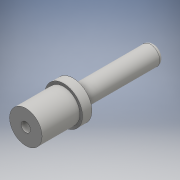
# Autodesk Inventor part: driven_shaft
Saved by Autodesk Inventor 2016 (Build 200138000, 138)
## iProperties
Created: 2015-10-28
Part Number: driven_shaft
Material: Gold
Document SubType Name: Modeling
Designer: Meet
Density: 19.3 g/cm^3
Appearance: Metal 1600F Hot
Author: Meet
Autodesk Inventor part; units mm, degrees
ref_plane "YZ Plane" through (0, 0, 0) normal (1, 0, 0) x (0, 1, 0)
ref_plane "XZ Plane" through (0, 0, 0) normal (0, 1, 0) x (-1, 0, 0)
ref_plane "XY Plane" through (0, 0, 0) normal (0, 0, 1) x (1, 0, 0)
sketch "Sketch1" plane through (0, 0, 0) normal (0, 1, 0) x (-1, 0, 0)
  circle A0 centre (0, 0) radius 10
  circle A1 centre (0, 0) radius 8.6
  constraints: 2 centre point, 2 coincident
extrude "Extrusion1" add sketch "Sketch1" along normal blind 5 contours A0 | A1
sketch "Sketch2" plane through (0, 0, 0) normal (0, -1, 0) x (1, 0, 0)
  circle A0 centre (0, 0) radius 8.6
  circle A1 centre (0, 0) radius 2.5
  constraints: 2 centre point, 2 coincident
extrude "Extrusion2" add sketch "Sketch2" along normal blind 20 contours A0 | A1
sketch "Sketch3" plane through (0, -20, 0) normal (0, -1, 0) x (1, 0, 0)
  circle A0 centre (0, 0) radius 2.5
  constraints: 1 centre point, 1 coincident
extrude "Extrusion3" cut sketch "Sketch3" against normal blind 10
sketch "Sketch4" plane through (0, 5, 0) normal (0, 1, 0) x (1, 0, 0)
  circle A0 centre (0, 0) radius 5
  constraints: 1 centre point
extrude "Extrusion4" add sketch "Sketch4" along normal blind 43
fillet "Fillet1" radius 2 1 edges at (-5, 48, 0)
body "Solid1"
